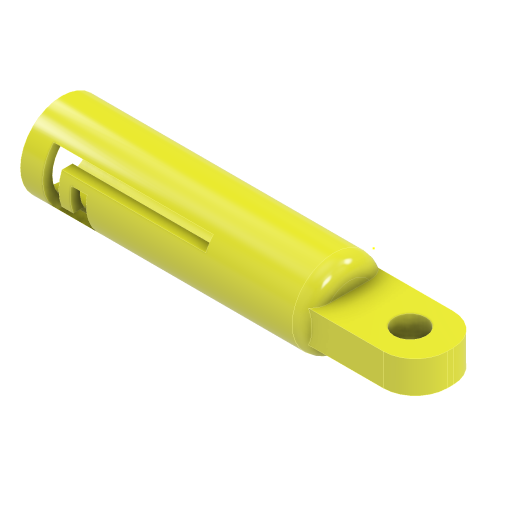
# Autodesk Inventor part: asteoscila1_(306)
Saved by Autodesk Inventor 2024 (Build 280153000, 153)
## iProperties
Created: 2024-04-19
Part Number: asteoscila1_(306)
Material: Generico
Document SubType Name: Modeling
Designer: Kelly
Density: 1 g/cm^3
Appearance: Giallo
Author: Kelly
Autodesk Inventor part; units mm, degrees
ref_plane "YZ Plane" through (0, 0, 0) normal (1, 0, 0) x (0, 1, 0)
sketch "Schizzo1" plane through (0, 0, 0) normal (0, 1, 0) x (-1, 0, 0)
  line L0 (0, 0) -> (0, -30)
  line L1 (0, -15) -> (90, -15)
  line L2 (100, 0) -> (100, -30)
  line L3 (0, -30) -> (100, -30)
  line L4 (100, 0) -> (0, 0)
  line L5 (100, -41.4573) -> (75, -41.4573)
  line L6 (75, -17) -> (85, -17)
  line L7 (75, -17) -> (75, -22)
  line L8 (85, -17) -> (85, -29.5)
  line L9 (75, -22) -> (80, -22)
  line L10 (80, -22) -> (80, -24.5)
  line L11 (80, -24.5) -> (5, -24.5)
  line L12 (85, -29.5) -> (5, -29.5)
  line L13 (5, -24.5) -> (5, -29.5)
  dimension "d0" = 30
  dimension "d1" = 90
  dimension "d5" = 25
  dimension "d6" = 17
  dimension "d7" = 10
  dimension "d8" = 5
  dimension "d9" = 12.5
  dimension "d10" = 5
  dimension "d11" = 2.5
  dimension "d13" = 80
  dimension "d16" = 75
  dimension "d76" = 100
  constraints: 28 end point, 7 horizontal, 5 vertical, 1 midpoint, 1 perpendicular, 1 other
  measures "d0" distance of L0.start L0.end
  measures "d1" distance of L1.start L1.end
  measures "d5" distance of L5.start L5.end
  measures "d6" distance between parallel lines of L4 L6
  measures "d7" distance of L6.start L6.end
  measures "d8" distance of L6.start L7.end
  measures "d9" distance of L6.end L8.end
  measures "d10" distance of L7.end L9.end
  measures "d11" distance of L9.end L10.end
  measures "d13" distance of L8.end L12.end
  measures "d16" distance of L10.end L11.end
  measures "d76" distance of L0.end L2.end
sketch "Schizzo2" plane through (0, 0, 0) normal (1, 0, 0) x (0, 1, 0)
  circle A0 centre (0, -15) radius 13
  circle A1 centre (0, -15) radius 12
  line L0 (5, -4.0913) -> (-5, -4.0913)
  line L1 (-5, -4.0913) -> (-5, -25.9087)
  line L2 (-5, -25.9087) -> (5, -25.9087)
  line L3 (5, -25.9087) -> (5, -4.0913)
  point P0 (0, 0)
  dimension "d2" = 15
  dimension "d3" = 26
  dimension "d53" = 24
  dimension "d58" = 10
  dimension "d59" = 21.8174
  constraints: 8 end point, 3 point on circle, 2 centre point, 2 parallel, 1 coincident, 1 horizontal, 1 perpendicular
  measures "d2" distance of point (0, 0) A0.centre
  measures "d3" diameter of A0
  measures "d53" diameter of A1
  measures "d58" distance of L0.start L0.end
  measures "d59" distance of L0.end L1.end
ref_plane "Piano di lavoro1" through (-90, 0, -15) normal (-1, 0, 0) x (0, -1, 0)
sketch "Schizzo3" plane through (-90, 0, -15) normal (-1, 0, 0) x (0, -1, 0)
  circle A0 centre (0, 0) radius 13
  point P0 (0, 15)
  dimension "d4" = 26
  constraints: 1 centre point
  measures "d4" diameter of A0
loft "Loft1" add profiles "Schizzo3", "Schizzo2" contours all / A0 | A1 L3 | L0 A1 | L3 L2 L1 L0 | A1 L2 | L1 A1
shell "Svuotamento1" thickness 3 removed faces 2 at (0, 3.4665, -13.963) at (-90, -3.4665, -13.963)
ref_plane "Piano di lavoro3" through (0, 0, -30) normal (0, 0.4988877, -0.8666667) x (-1, 0, 0)
sketch "Schizzo11" plane through (0, 0, -30) normal (0, 0.4988877, -0.8666667) x (-1, 0, 0)
  point P0 (0, 14.9666)
extrude "Estrusione5" add sketch "Schizzo2" against normal blind 10 contours A1 L3 | L0 A1 | L3 L2 L1 L0 | A1 L2 | L1 A1
extrude "Estrusione6" add sketch "Schizzo2" along normal blind 31.4 contours L3 L2 L1 L0
fillet "Raccordo1" radius 10 1 edges at (31.4, 0, -25.9087)
fillet "Raccordo2" radius 10 1 edges at (31.4, 0, -4.0913)
sketch "Schizzo12" plane through (0, -5, -25.9087) normal (0, -1, 0) x (1, 0, 0)
  line L0 (0, 0) -> (21.4, 0) projected
  line L1 (6.4, 21.8172) -> (21.4, 21.8172)
  line L2 (31.4, 11.8174) -> (31.4, 10) projected
  circle A0 centre (18.9, 10.9087) radius 5
  line L3 (0, 25.9087) -> (0, -2.0913) projected
  point P0 (13.9, 21.8172)
  point P1 (31.4, 10.9087)
  point P2 (10.7, 0)
  point P3 (31.4, 10.9087)
  point P4 (0, -2.0913)
  dimension "d64" = 21.8172
  dimension "d70" = 10
  dimension "d71" = 12.5
  dimension "d72" = 10.9085
  dimension "d75" = 18.9
  constraints: 4 midpoint, 2 end point, 1 centre point, 1 other
  measures "d64" distance from line of L0 point (13.9, 21.817)
  measures "d70" diameter of A0
  measures "d71" distance of point (31.4, 10.909) A0.centre
  measures "d72" distance from line of L1 A0.centre
extrude "Estrusione7" cut sketch "Schizzo12" against normal blind 25
fillet "Raccordo3" radius 5 1 edges at (0, 13, -15)
sketch "Schizzo13" plane through (0, 0, 0) normal (0, 0, 1) x (1, 0, 0)
  line L0 (-33, 8.7721) -> (-83, 8.7721)
  line L1 (-90, 10) -> (-10, 10) projected
  line L2 (-33, 8.7721) -> (-33, 5)
  line L3 (-5, -13) -> (-5, 13) projected
  line L4 (-83, 8.7721) -> (-83, -10)
  line L5 (-83, -10) -> (-69.4203, -10)
  line L6 (-90, -10) -> (-10, -10) projected
  line L7 (-69.4203, -10) -> (-69.4203, 2.7972)
  line L8 (-69.4203, 2.7972) -> (-74.4203, 2.7972)
  line L9 (-74.4203, 2.7972) -> (-74.4203, -5)
  line L10 (-74.4203, -5) -> (-78, -5)
  line L11 (-78, -5) -> (-78, 5)
  line L12 (-33, 5) -> (-78, 5)
  point P0 (0, 0)
  point P1 (-33, 6.8861)
  dimension "d21" = 3
  dimension "d79" = 28
  dimension "d80" = 50
  dimension "d83" = 5
  dimension "d84" = 5
  dimension "d85" = 7.7972
  dimension "d86" = 5
  dimension "d87" = 5
  constraints: 20 end point, 4 perpendicular, 3 vertical, 1 horizontal, 1 midpoint, 1 point on line
  measures "d79" distance from line of point (-33, 6.886) L3
  measures "d80" distance of L0.start L0.end
  measures "d83" distance between parallel lines of L12 L1
  measures "d84" distance between parallel lines of L9 L7
  measures "d85" distance of L8.end L9.end
  measures "d86" distance between parallel lines of L4 L11
  measures "d87" distance between parallel lines of L6 L10
extrude "Estrusione8" cut sketch "Schizzo13" against normal blind 10
